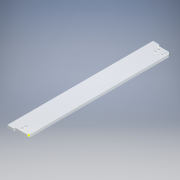
# Autodesk Inventor part: X_Kettenhalter
Saved by Autodesk Inventor 2021.3 (Build 253353000, 353)
## iProperties
Created: 2021-04-26
Part Number: X_Kettenhalter
Material: Generic
Document SubType Name: Modeling
Designer: Fabijan_Sven
Density: 1 g/cm^3
Appearance: Clear
Author: Fabijan_Sven
Autodesk Inventor part; units mm, degrees
ref_plane "YZ Plane" through (0, 0, 0) normal (1, 0, 0) x (0, 1, 0)
ref_plane "XZ Plane" through (0, 0, 0) normal (0, 1, 0) x (-1, 0, 0)
ref_plane "XY Plane" through (0, 0, 0) normal (0, 0, 1) x (1, 0, 0)
sketch "Sketch1" plane through (0, 0, 0) normal (0, 1, 0) x (-1, 0, 0)
  line L0 (0, 0) -> (62, 0)
  line L1 (62, 0) -> (62, -450)
  line L2 (62, -450) -> (0, -450)
  line L3 (0, -450) -> (0, 0)
  dimension "d0" = 62
  dimension "d1" = 450
  constraints: 8 end point, 2 parallel, 1 horizontal, 1 perpendicular
  measures "d0" distance of L1.end L2.end
  measures "d1" distance of L0.end L1.end
extrude "Extrusion1" add sketch "Sketch1" along normal blind 8
fillet "Fillet1" radius 10 2 edges at (0, 4, 0) (0, 4, -450)
sketch "Sketch3" plane through (0, 8, 0) normal (0, 1, 0) x (1, 0, 0)
  point P0 (0, 0)
sketch "Sketch4" plane through (0, 8, 0) normal (0, 1, 0) x (1, 0, 0)
  circle A0 centre (-10, 440) radius 2
  circle A1 centre (-10, 432) radius 2
  line L0 (0, 10) -> (0, 440) projected
  line L1 (-10, 450) -> (-62, 450) projected
  point P0 (0, 0)
  dimension "d25" = 10
  dimension "d26" = 10
  dimension "d27" = 4
  dimension "d28" = 4
  dimension "d29" = 10
  dimension "d30" = 8
  constraints: 2 centre point
  measures "d25" distance from line of L0 A0.centre
  measures "d26" distance from line of L0 A1.centre
  measures "d27" diameter of A1
  measures "d28" diameter of A0
  measures "d29" distance from line of L1 A0.centre
  measures "d30" distance of A0.centre A1.centre
hole "Hole2" at (-10, 8, -432) at (-10, 8, -440) direction (0, -1, 0) diameter 4 end through all
sketch "Sketch5" plane through (0, 8, 0) normal (0, 1, 0) x (1, 0, 0)
  point P0 (0, 0)
sketch "Sketch6" plane through (0, 8, 0) normal (0, 1, 0) x (1, 0, 0)
  circle A0 centre (-30, 20) radius 2.6
  circle A1 centre (-30, 10) radius 2.6
  line L0 (-62, 0) -> (-10, 0) projected
  line L1 (-62, 450) -> (-62, 0) projected
  line L2 (-101.8296, 225) -> (129.7674, 225) construction
  circle A2 centre (-30, 430) radius 2.6
  circle A3 centre (-30, 440) radius 2.6
  point P0 (0, 0)
  point P1 (-10, 450)
  dimension "d38" = 5.2
  dimension "d39" = 5.2
  dimension "d40" = 20
  dimension "d41" = 10
  dimension "d42" = 32
  dimension "d43" = 32
  dimension "d44" = 225
  constraints: 4 centre point, 3 symmetric about line, 2 end point, 1 horizontal, 2 other
  measures "d38" diameter of A1
  measures "d39" diameter of A0
  measures "d40" distance from line of L0 A0.centre
  measures "d41" distance from line of L0 A1.centre
  measures "d42" distance from line of A1.centre L1
  measures "d43" distance from line of L1 A0.centre
  measures "d44" distance between parallel lines of L2 L0
hole "Hole3" at (-30, 8, -20) at (-30, 8, -10) at (-30, 8, -440) at (-30, 8, -430) direction (0, -1, 0) diameter 5.2 end through all
sketch "Sketch7" plane through (0, 8, 0) normal (0, 1, 0) x (1, 0, 0)
  line L0 (-62, 450) -> (-62, 0) projected
  line L1 (-62, 0) -> (-42, 0)
  line L2 (-42, 0) -> (-42, -5)
  line L3 (-42, -5) -> (-62, -5)
  line L4 (-62, -5) -> (-62, 0)
  line L5 (-62, 450) -> (-42, 450)
  line L6 (-42, 450) -> (-42, 455)
  line L7 (-42, 455) -> (-62, 455)
  line L8 (-62, 455) -> (-62, 450)
  point P0 (0, 0)
  dimension "d52" = 20
  dimension "d53" = 5
  dimension "d54" = 20
  dimension "d55" = 5
  constraints: 16 end point, 4 parallel, 2 horizontal, 2 perpendicular
  measures "d52" distance of L2.end L3.end
  measures "d53" distance of L3.end L0.end
  measures "d54" distance of L6.end L7.end
  measures "d55" distance of L5.end L6.end
extrude "Extrusion2" add sketch "Sketch7" against normal blind 8
equation "\"d31\" = d28"
body "Solid1"
